# Autodesk Inventor part: 同步皮带
Saved by Autodesk Inventor 2015 (Build 190159000, 159)
## iProperties
Created: 2017-05-28
Part Number: 同步皮带
Material: Rubber
Document SubType Name: Modeling
Designer: Administrator
Density: 1 g/cm^3
Appearance: Rubber - Black - Version 1.1
CustomPartVersion: 1
Author: Administrator
Autodesk Inventor part; units mm, degrees
sketch "草图路径" plane through (0, 0, 0) normal (0, 0, 1) x (1, 0, 0)
  arc A0 (-0.6145, 24.2474) -> (-21.4612, -11.3019) centre (0, 0) ccw
  arc A1 (255.7542, -161.4167) -> (270.1959, 31.1107) centre (272.654, -65.879) ccw
  arc A2 (31.7001, -112.2498) -> (48.9363, -124.8323) centre (53.1612, -100.9479) ccw
  line L0 (31.7001, -112.2498) -> (-21.4612, -11.3019)
  line L1 (-0.6145, 24.2474) -> (270.1959, 31.1107)
  line L2 (255.7542, -161.4167) -> (48.9363, -124.8323)
  constraints: 6 end point, 6 point on circle, 3 centre point
ref_plane "截面平面" through (-21.4612, -11.3019, 0) normal (0.466, -0.8848, 0) x (0, 0, 1)
ref_plane "工作平面2" through (0, 0, 0) normal (-1, 0, 0) x (0, 0, 1)
ref_plane "工作平面3" through (272.654, -65.879, 0) normal (-0.9976, 0.0686, 0) x (0, 0, 1)
ref_plane "工作平面4" through (53.1612, -100.9479, 0) normal (0.8703, -0.4925, 0) x (0, 0, 1)
sketch "截面" plane through (-21.4612, -11.3019, 0) normal (0.466, -0.8848, 0) x (0, 0, 1)
  line L0 (-9.525, 1.3462) -> (9.525, 1.3462)
  line L1 (9.525, 1.3462) -> (9.525, -0.6858)
  line L2 (9.525, -0.6858) -> (-9.525, -0.6858)
  line L3 (-9.525, -0.6858) -> (-9.525, 1.3462)
  line L4 (-9.525, 0) -> (9.525, 0) construction
  point P0 (0, 0)
  point P1 (0, 0)
  dimension "d0" = 19.05
  dimension "d4" = 0.6858
  dimension "d5" = 1.3462
  constraints: 10 end point, 2 parallel, 2 point on line, 1 coincident, 1 horizontal, 1 midpoint, 1 perpendicular, 1 other
  measures "d0" distance between parallel lines of L1 L3
  measures "d4" distance between parallel lines of L2 L4
  measures "d5" distance between parallel lines of L4 L0
sweep "皮带" add profiles "截面" path "草图路径"
equation "\"d0\" = da_B"
equation "\"d4\" = da_a"
equation "\"d5\" = da_a2"
equation "\"da_B\" = 19.05"
equation "\"da_pb\" = 12.7"
equation "\"da_L\" = 990.6"
equation "\"da_a\" = 0.6858"
equation "\"da_S\" = 6.1214"
equation "\"da_Beta\" = 20deg"
equation "\"da_Ht\" = 2.286"
equation "\"da_H\" = 4.318"
equation "\"da_a2\" = 1.3462"
body "Solid1"
